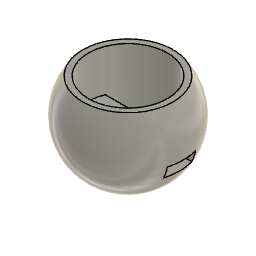
Owl_head_v9 (Autodesk Fusion 360 design; units mm, degrees)
Autodesk Fusion 360 part; units mm, degrees
sketch "Esquisse1" plane through (0, 0, 0) normal (0, 0, 1) x (1, 0, 0)
sphere "SpherePrimitive1" add diameter 100 placed x (1, 0, 0) y (0, 1, 0) z (0, 0, 1) at (20, 20, 0) makes body 1
sketch "Esquisse3" plane through (0, 0, 0) normal (0, 0, 1) x (1, 0, 0)
ref_plane "Plan de construction1" through (0, 0, 30) normal (0, 0, 1) x (1, 0, 0)
sketch "Esquisse4" plane through (0, 0, 30) normal (0, 0, 1) x (1, 0, 0)
  circle A0 centre (20, 20) radius 40
  dimension "d3" = 80
  measures "d3" diameter of A0
extrude "Extrusion1" cut sketch "Esquisse4" along normal through all bodies 1
sketch "Esquisse5" plane through (0, 0, 30) normal (0, 0, 1) x (-1, 0, 0)
  circle A0 centre (-20, -20) radius 40
  circle A1 centre (-20, -20) radius 35
  dimension "d5" = 70
  constraint concentric A0 A1
  measures "d5" diameter of A1
extrude "Extrusion2" cut sketch "Esquisse5" against normal blind 60 contours A1 bodies 1
copy_body "Corps->Comp1" bodies 1 removing the originals makes body 2 in component "head"
ref_plane "Plan de construction2" through (20, 20, -10) normal (0, 0, 1) x (1, 0, 0)
sketch "Esquisse7" plane through (20, 20, -10) normal (0, 0, 1) x (1, 0, 0)
  line L0 (55, 12.5003) -> (10, 12.5003)
  line L1 (10, 12.5003) -> (10, -12.4997)
  line L2 (10, -12.4997) -> (55, -12.4997)
  line L3 (55, -12.4997) -> (55, 12.5003)
  line L4 (-55, -12.5379) -> (-10, -12.5379)
  line L5 (-10, -12.5379) -> (-10, 12.4621)
  line L6 (-10, 12.4621) -> (-55, 12.4621)
  line L7 (-55, 12.4621) -> (-55, -12.5379)
  line L8 (10, -12.4997) -> (10, 12.5003)
  line L9 (10, 12.5003) -> (32.5, 12.5003)
  line L10 (10, -12.4997) -> (32.5, -12.4997)
  line L11 (10, 12.5003) -> (32.5, 12.5003)
  line L12 (-10, -12.5379) -> (-32.5, -12.5379)
  line L13 (-10, 12.4621) -> (-32.5, 12.4621)
  arc A0 (32.5, -12.4997) -> (32.5, 12.5003) centre (2.5, 0.0003) ccw
  arc A1 (-32.5, 12.4621) -> (-32.5, -12.5379) centre (-2.5003, -0.0379) ccw
  point P0 (-10, 12.4621)
  point P1 (10, 0.0003)
  point P2 (-10, -0.0379)
  dimension "d9" = 45
  dimension "d10" = 25
  dimension "d11" = 45
  dimension "d12" = 25
  dimension "d14" = 12.5
  dimension "d15" = 10
  dimension "d16" = 10
  constraint horizontal L0
  constraint vertical L1
  constraint horizontal L2
  constraint vertical L3
  constraint horizontal L4
  constraint vertical L5
  constraint horizontal L6
  constraint vertical L7
  constraint coincident P0 L5.end
  constraint coincident L0 L9.end
  constraint midpoint L2 L10.end
  constraint midpoint L0 L9.end
  constraint midpoint L4 L12.end
  constraint midpoint L6 L13.end
  constraint midpoint L1 P1
  constraint midpoint L5 P2
  measures "d9" distance of L0.start L0.end
  measures "d10" distance of L0.end L1.end
  measures "d11" distance of P0 L6.end
  measures "d12" distance of L4.end P0
  measures "d14" distance of L1.end P1
  measures "d15" distance of origin L5
  measures "d16" distance of origin L8
extrude "Extrusion1'" add sketch "Esquisse7" along normal blind 3 contours L0 L1 L2 L8 L9 L10 L11 A0 | L4 L5 L6 L12 L13 A1 bodies 2 in component "head"
sketch "Esquisse8" plane through (0, 0, -9.5651) normal (0, 0, -1) x (1, 0, 0)
  line L0 (51.9972, -7.6484) -> (29.4972, -7.6484)
  line L1 (29.4972, -7.6484) -> (29.4972, -32.6484)
  line L2 (29.4972, -32.6484) -> (51.9972, -32.6484)
  arc A0 (51.9972, -32.6484) -> (54.4972, -20.1517) centre (21.9972, -20.1484) ccw
  arc A1 (54.4972, -20.1517) -> (51.9972, -7.6484) centre (21.9972, -20.1484) ccw
  line L3 (-13.3, -32.6) -> (-35.8, -32.6)
  line L4 (-35.8, -32.6) -> (-35.8, -7.6)
  line L5 (-35.8, -7.6) -> (-13.3, -7.6)
  line L6 (-13.3, -7.6) -> (-13.3, -32.6)
  line L7 (51.9972, -32.6484) -> (74.4972, -32.6484)
  line L8 (74.4972, -32.6484) -> (74.4972, -7.6484)
  line L9 (74.4972, -7.6484) -> (51.9972, -7.6484)
  line L10 (51.9972, -7.6484) -> (51.9972, -32.6484)
  dimension "d19" = 25
  dimension "d20" = 22.5
  dimension "d21" = 22.5
  constraint horizontal L3
  constraint vertical L4
  constraint horizontal L5
  constraint vertical L6
  constraint horizontal L7
  constraint vertical L8
  constraint horizontal L9
  constraint vertical L10
  constraint coincident L2.end A0.start
  measures "d19" distance of L3.start L5.end
  measures "d20" distance of L3.start L3.end
  measures "d21" distance of L8.end L0.start
extrude "Extrusion2'" cut sketch "Esquisse8" along normal blind 10 contours A0 A1 L7 L8 L9 | L3 L4 L5 L6 sketch seen with x (1, 0, 0) y (0, 1, 0) z (0, 0, 1) at (0.5028, -0.1481, -0.4349) bodies 2 in component "head"
component "head" placed x (1, 0, 0) y (0, 1, 0) z (0, 0, 1) at (-0.5028, 0.1481, 0.4349)
named bodies: "head"
